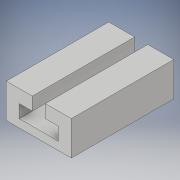
# Autodesk Inventor part: testrail
Saved by Autodesk Inventor 2018 (Build 220112000, 112)
## iProperties
Created: 2018-04-30
Part Number: testrail
Material: Generic
Document SubType Name: Modeling
Designer: 4070609
Density: 1 g/cm^3
Appearance: Default
Author: 4070609
Autodesk Inventor part; units mm, degrees
ref_plane "YZ Plane" through (0, 0, 0) normal (1, 0, 0) x (0, 1, 0)
ref_plane "XZ Plane" through (0, 0, 0) normal (0, 1, 0) x (-1, 0, 0)
ref_plane "XY Plane" through (0, 0, 0) normal (0, 0, 1) x (1, 0, 0)
sketch "Sketch1" plane through (0, 0, 0) normal (0, 1, 0) x (-1, 0, 0)
  line L0 (0, 0) -> (16, 0)
  line L1 (16, 0) -> (16, -25.2)
  line L2 (16, -25.2) -> (0, -25.2)
  line L3 (0, -25.2) -> (0, 0)
  dimension "d0" = 16
  dimension "d1" = 25.2
  constraints: 8 end point, 2 parallel, 1 horizontal, 1 perpendicular
  measures "d0" distance of L1.end L2.end
  measures "d1" distance of L0.end L1.end
extrude "Extrusion1" add sketch "Sketch1" along normal blind 2
sketch "Sketch2" plane through (-16, 0, 0) normal (0, 0, 1) x (1, 0, 0)
  line L0 (0, 2) -> (16, 2) projected
  line L1 (16, 2) -> (16, 8.4)
  line L2 (16, 8.4) -> (9.6, 8.4)
  line L3 (9.6, 8.4) -> (9.6, 5.2)
  line L4 (9.6, 5.2) -> (12.8, 5.2)
  line L5 (12.8, 5.2) -> (12.8, 2)
  line L6 (12.8, 2) -> (16, 2)
  line L7 (0, 2) -> (0, 8.4)
  line L8 (0, 8.4) -> (6.4, 8.4)
  line L9 (6.4, 8.4) -> (6.4, 5.2)
  line L10 (6.4, 5.2) -> (3.2, 5.2)
  line L11 (3.2, 5.2) -> (3.2, 2)
  point P0 (16, 0)
  dimension "d4" = 6.4
  dimension "d5" = 6.4
  dimension "d6" = 3.2
  dimension "d7" = 3.2
  dimension "d8" = 6.4
  dimension "d9" = 3.2
  constraints: 22 end point, 5 perpendicular, 3 horizontal, 2 point on line, 2 vertical, 1 collinear
  measures "d4" distance of L0.end L1.end
  measures "d5" distance of L1.end L2.end
  measures "d6" distance of L2.end L3.end
  measures "d7" distance of L3.end L4.end
  measures "d8" distance of L7.end L8.end
  measures "d9" distance of L8.end L9.end
extrude "Extrusion2" add sketch "Sketch2" against normal blind 25.2
body "Solid1"
